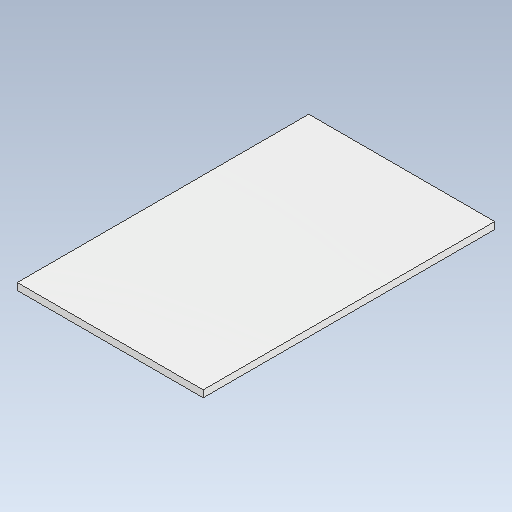
# Autodesk Inventor part: pokrywa_obudowy_elektroniki
Saved by Autodesk Inventor 2020 (Build 240168000, 168)
## iProperties
Created: 2020-08-31
Part Number: pokrywa_obudowy_elektroniki
Material: ABS Plastic
Document SubType Name: Modeling
Designer: Hesekiel
Density: 1.06 g/cm^3
Appearance: Smooth - White
Mass: 32.7127 g
Surface Area: 218.22 cm^2
Volume: 30.861 cm^3
Author: Hesekiel
Autodesk Inventor part; units mm, degrees
ref_plane "YZ Plane" through (0, 0, 0) normal (1, 0, 0) x (0, 1, 0)
ref_plane "XZ Plane" through (0, 0, 0) normal (0, 1, 0) x (-1, 0, 0)
ref_plane "XY Plane" through (0, 0, 0) normal (0, 0, 1) x (1, 0, 0)
sketch "Sketch1" plane through (0, 0, 0) normal (0, 1, 0) x (-1, 0, 0)
  line L0 (-40.5, 63.5) -> (40.5, 63.5)
  line L1 (40.5, 63.5) -> (40.5, -63.5)
  line L2 (40.5, -63.5) -> (-40.5, -63.5)
  line L3 (-40.5, -63.5) -> (-40.5, 63.5)
  line L4 (-40.5, 63.5) -> (40.5, -63.5) construction
  line L5 (40.5, 63.5) -> (-40.5, -63.5) construction
  point P0 (0, 0)
  dimension "d0" = 81
  dimension "d1" = 127
  constraints: 12 end point, 2 midpoint, 2 parallel, 1 horizontal, 1 perpendicular
  measures "d0" distance of L1.end L2.end
  measures "d1" distance of L0.end L1.end
extrude "Extrusion1" add sketch "Sketch1" along normal blind 3
body "Solid1"
